Autodesk Fusion 360 part; units mm, degrees
(part 2 of 2)
sketch "Sketch44" plane through (-35.5, 0, 0) normal (-1, 0, 0) x (0, -1, 0)
  line L0 (-45.15, 0.15) -> (-50.15, 0.15)
  line L1 (-50.15, 0.15) -> (-50.15, -5.15)
  line L2 (-50.15, -5.15) -> (-33.85, -5.15)
  line L3 (-33.85, -5.15) -> (-33.85, 0.15)
  line L4 (-33.85, 0.15) -> (-38.85, 0.15)
  line L5 (-38.85, 0.15) -> (-38.85, 35.15)
  line L6 (-38.85, 35.15) -> (-40.65, 35.15)
  line L7 (-40.65, 35.15) -> (-40.65, 30.15)
  line L8 (-40.65, 30.15) -> (-43.35, 30.15)
  line L9 (-43.35, 30.15) -> (-43.35, 35.15)
  line L10 (-43.35, 35.15) -> (-45.15, 35.15)
  line L11 (-45.15, 35.15) -> (-45.15, 0.15)
extrude "Extrude51" add sketch "Sketch32" along normal blind 1 separate body makes body 28
sketch "Sketch45" plane through (0, 39.5, 0) normal (0, -1, 0) x (1, 0, 0)
  line L0 (-33, 68.5049) -> (-47.2038, 22.85)
  line L1 (-47.2038, 22.85) -> (-34.35, 22.85)
  line L2 (-34.35, 22.85) -> (-34.35, 34.85)
  line L3 (-34.35, 34.85) -> (-31.65, 34.85)
  line L4 (-31.65, 34.85) -> (-31.65, 22.85)
  line L5 (-31.65, 22.85) -> (-18.7962, 22.85)
  line L6 (-18.7962, 22.85) -> (-33, 68.5049)
extrude "Extrude52" add sketch "Sketch33" along normal blind 1 separate body makes body 29
sketch "Sketch46" plane through (2.5, 0, 0) normal (-1, 0, 0) x (0, -1, 0)
  line L0 (-37.85, 23.15) -> (-39.65, 23.15)
  line L1 (-39.65, 23.15) -> (-39.65, 18.15)
  line L2 (-39.65, 18.15) -> (-42.35, 18.15)
  line L3 (-42.35, 18.15) -> (-42.35, 23.15)
  line L4 (-42.35, 23.15) -> (-44.15, 23.15)
  line L5 (-44.15, 23.15) -> (-44.15, 0.15)
  line L6 (-44.15, 0.15) -> (-49.15, 0.15)
  line L7 (-49.15, 0.15) -> (-49.15, -5.15)
  line L8 (-49.15, -5.15) -> (-32.85, -5.15)
  line L9 (-32.85, -5.15) -> (-32.85, 0.15)
  line L10 (-32.85, 0.15) -> (-37.85, 0.15)
  line L11 (-37.85, 0.15) -> (-37.85, 23.15)
extrude "Extrude53" add sketch "Sketch34" along normal blind 1 separate body makes body 30
sketch "Sketch47" plane through (0, 38.5, 0) normal (0, -1, 0) x (1, 0, 0)
  line L0 (-5.2005, 10.85) -> (3.65, 10.85)
  line L1 (3.65, 10.85) -> (3.65, 22.85)
  line L2 (3.65, 22.85) -> (6.35, 22.85)
  line L3 (6.35, 22.85) -> (6.35, 10.85)
  line L4 (6.35, 10.85) -> (15.2005, 10.85)
  line L5 (15.2005, 10.85) -> (5, 45.5316)
  line L6 (5, 45.5316) -> (-5.2005, 10.85)
equation "d4 = material"
equation "d6 = material"
equation "d17 = material"
equation "d19 = -material"
equation "d25 = -material"
equation "d29 = material"
equation "d33 = material"
equation "material = 3 mm"
equation "kerf = 0.15 mm"
equation "d37 = -material"
equation "d47 = material"
equation "d49 = material"
equation "d50 = material"
equation "d52 = material"
equation "d53 = material"
equation "d63 = material"
equation "d65 = -material"
equation "d68 = material"
equation "d78 = material"
equation "d80 = -material"
equation "d83 = material"
equation "d93 = material"
equation "d95 = -material"
equation "d98 = material"
equation "d108 = material"
equation "d110 = -material"
equation "d113 = material"
equation "d115 = -material"
equation "d117 = -material"
equation "d119 = kerf"
equation "d120 = kerf"
equation "d121 = kerf"
equation "d122 = kerf"
equation "d123 = kerf"
equation "d124 = kerf"
equation "d125 = kerf"
equation "d126 = kerf"
equation "d127 = kerf"
equation "d128 = kerf"
equation "d129 = kerf"
equation "d130 = kerf"
equation "d131 = kerf"
equation "d132 = kerf"
equation "d133 = kerf"
equation "d134 = kerf"
equation "d135 = kerf"
equation "d136 = kerf"
equation "d137 = kerf"
equation "d138 = kerf"
equation "d139 = kerf"
equation "d140 = kerf"
named bodies: "Base", "LeftLeg", "RightLeg", "FrontPlate", "Trunk1", "Leafs1", "Trunk2", "Leafs2", "Trunk3", "Leafs3", "Trunk4", "Leafs4", "Trunk5"
